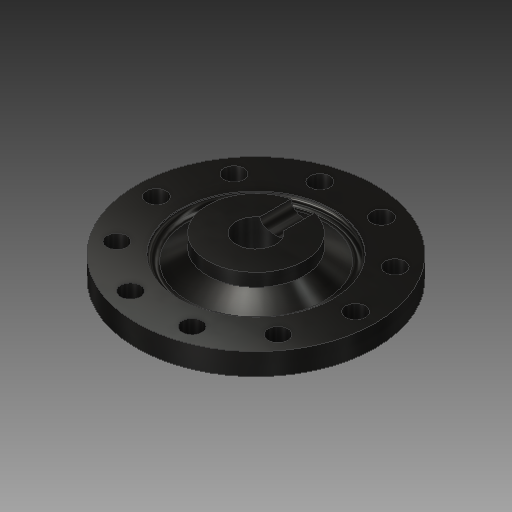
# Autodesk Inventor part: 212-04
Saved by Autodesk Inventor 2019 (Build 230136000, 136)
## iProperties
Company: Autodesk Inc.
Created: 2017-03-14
Part Number: 212-04
Material: Steel, Alloy
Document SubType Name: Modeling
Designer: Autodesk Inc.
Density: 7.73 g/cm^3
Appearance: Anodized - Subtle Dark Bronze Satin
Mass: 117.111 g
Surface Area: 78.0055 cm^2
Volume: 15.1502 cm^3
Author: Inventor
Autodesk Inventor part; units mm, degrees
ref_plane "YZ Plane" through (0, 0, 0) normal (1, 0, 0) x (0, 1, 0)
ref_plane "XZ Plane" through (0, 0, 0) normal (0, 1, 0) x (-1, 0, 0)
ref_plane "XY Plane" through (0, 0, 0) normal (0, 0, 1) x (1, 0, 0)
sketch "Sketch1" plane through (0, 0, 0) normal (0, 0, 1) x (1, 0, 0)
  line L0 (30, 0) -> (30, 5.439)
  line L1 (30, 5.439) -> (19.392, 5.439)
  line L2 (19.392, 5.439) -> (19.392, 2.5321)
  line L3 (12.155, 10.043) -> (0, 10.043)
  line L4 (0, 10.043) -> (0, 0)
  line L5 (0, 0) -> (30, 0)
  line L6 (12.155, 10.043) -> (12.155, 6.812)
  line L7 (12.155, 6.812) -> (19.392, 2.5321)
  dimension "d1" = 30
  dimension "d2" = 10.043
  dimension "d3" = 5.439
  dimension "d4" = 10.608
  dimension "d5" = 3.231
  dimension "d6" = 120.6
  dimension "d7" = 17.845
  constraints: 16 end point, 3 perpendicular, 3 vertical, 1 parallel
  measures "d1" distance of L4.end L0.start
  measures "d2" distance of L3.end L4.end
  measures "d3" distance of L0.start L0.end
  measures "d4" distance between parallel lines of L0 L2
  measures "d5" distance of L3.start L6.end
  measures "d6" angle of L6 L7
  measures "d7" distance between parallel lines of L0 L6
revolve "Revolution1" add sketch "Sketch1" angle 360 about axis through (0, 10.043, 0) along (0, -1, 0)
fillet "Fillet1" radius 1.5 1 edges at (-19.392, 2.5321, 0)
sketch "Sketch2" plane through (0, 0, 0) normal (0, -1, 0) x (1, 0, 0)
  circle A0 centre (0, 0) radius 30 projected
  point P0 (25, 0)
  dimension "d10" = 25
  constraints: 1 horizontal alignment
  measures "d10" distance of A0.centre point (25, 0)
hole "Hole1" at (25, 0, 0) direction (0, 1, 0) diameter 5 end through all
pattern_circular "Circular Pattern1" count 10 over 360 about axis through (0, -10, 0) along (0, 1, 0) of "Hole1"
sketch "Sketch3" plane through (0, 10.043, 0) normal (0, 1, 0) x (1, 0, 0)
  circle A0 centre (0, 0) radius 12.155 projected
hole "Hole2" at (0, 10.043, 0) direction (0, -1, 0) diameter 7.936 end through all counterbore diameter 9.938 counterbore depth 7.672
sketch "Sketch4" plane through (0, 0, 0) normal (0, 0, 1) x (1, 0, 0)
  line L0 (-12.155, 10.043) -> (12.155, 10.043) construction
  line L1 (0, -6.974) -> (0, 27.06) construction
  point P0 (0, 10.043)
  constraints: 2 midpoint
hole "Hole3" at (0, 10.043, 0) direction (0, 0, -1) diameter 6 end through all
body "Solid1"
